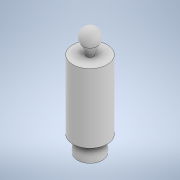
# Autodesk Inventor part: octopus tentacles
Saved by Autodesk Inventor 2022 (Build 260153000, 153)
## iProperties
Created: 2020-07-11
Part Number: octopus tentacles
Material: Generic
Document SubType Name: Modeling
Designer: saipr
Density: 1 g/cm^3
Appearance: Default
Mass: 6.74938 g
Surface Area: 24.3925 cm^2
Volume: 6.74938 cm^3
Author: saipr
Autodesk Inventor part; units mm, degrees
ref_plane "YZ Plane" through (0, 0, 0) normal (1, 0, 0) x (0, 1, 0)
ref_plane "XZ Plane" through (0, 0, 0) normal (0, 1, 0) x (-1, 0, 0)
ref_plane "XY Plane" through (0, 0, 0) normal (0, 0, 1) x (1, 0, 0)
sketch "Sketch2" plane through (0, 0, 0) normal (0, 0, 1) x (1, 0, 0)
  circle A0 centre (0, 0) radius 3.175
  line L0 (-6.35, -5.715) -> (6.35, -5.715)
  line L1 (6.35, -5.715) -> (6.35, -31.115)
  line L2 (6.35, -31.115) -> (-6.35, -31.115)
  line L3 (-6.35, -31.115) -> (-6.35, -5.715)
  line L4 (-6.35, -5.715) -> (6.35, -31.115) construction
  line L5 (6.35, -5.715) -> (-6.35, -31.115) construction
  line L6 (0, -3.175) -> (0, -5.715)
  line L7 (0, -5.715) -> (1.27, -5.715)
  line L8 (1.27, -5.715) -> (-1.27, -5.715)
  arc A1 (-1.27, -5.715) -> (-2.6064, -1.8131) centre (-8.7785, -6.1069) ccw
  arc A2 (2.5875, -1.84) -> (1.27, -5.715) centre (8.4115, -5.9816) ccw
  line L9 (0, -31.115) -> (0, -32.7025)
  arc A3 (4.5781, -37.1898) -> (-4.5781, -37.1898) centre (0, -35.8775) ccw
  arc A4 (2.8911, -37.1898) -> (-2.8911, -37.1898) centre (0, -35.8775) ccw
  line L10 (0, -31.115) -> (0, -36.703)
  line L11 (2.8911, -37.1898) -> (4.5781, -37.1898)
  line L12 (4.5781, -37.1898) -> (2.8911, -37.1898)
  line L13 (-2.8911, -37.1898) -> (-4.5781, -37.1898)
  line L14 (0, -32.7025) -> (0, 3.175)
  line L15 (2.6326, -31.9088) -> (2.6326, -31.115)
  line L16 (-2.6326, -31.9088) -> (-2.6326, -31.115)
  point P0 (0, -18.415)
  point P1 (0, -31.115)
  point P2 (0, -31.115)
  point P3 (0, -5.715)
  dimension "d25" = 6.35
  dimension "d27" = 12.7
  dimension "d28" = 25.4
  dimension "d29" = 2.54
  dimension "d30" = 1.27
  dimension "d31" = 2.54
  dimension "d34" = 5.588
  dimension "d36" = 4.7625
  dimension "d37" = 3.175
  constraints: 34 end point, 16 point on circle, 6 point on line, 5 centre point, 3 collinear, 3 horizontal, 3 midpoint, 3 perpendicular, 3 vertical, 2 coincident, 2 parallel, 2 tangent
  measures "d25" diameter of A0
  measures "d27" distance of L1.end L2.end
  measures "d28" distance of L0.end L1.end
  measures "d29" distance of L6.start L6.end
  measures "d30" distance of L6.end L7.end
  measures "d31" distance of L7.end L8.end
  measures "d34" distance of L9.start L10.end
  measures "d36" radius of A3
  measures "d37" radius of A4
revolve "Revolution2" add sketch "Sketch2" angle 360 about axis through (0, -32.7025, 0) along (0, 1, 0) picked at (1.1451, 0.9452) contours A0 L14 | A2 L0 L6 A0 | L0 L1 L2 L14 | A3 L11 A4 L9 | L2 L15 A3
body "Solid2"
